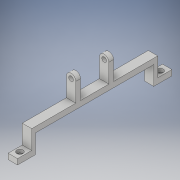
# Autodesk Inventor part: ventilador emergència inferior
Saved by Autodesk Inventor 2019 (Build 230136000, 136)
## iProperties
Created: 2018-10-29
Part Number: ventilador emergència inferior
Material: Genérico
Document SubType Name: Modeling
Designer: Albert Garangou Culebras
Density: 1 g/cm^3
Appearance: Valor por defecto
Author: Albert Garangou Culebras
Autodesk Inventor part; units mm, degrees
ref_plane "YZ Plane" through (0, 0, 0) normal (1, 0, 0) x (0, 1, 0)
ref_plane "XZ Plane" through (0, 0, 0) normal (0, 1, 0) x (-1, 0, 0)
ref_plane "XY Plane" through (0, 0, 0) normal (0, 0, 1) x (1, 0, 0)
sketch "Boceto1" plane through (0, 0, 0) normal (0, 1, 0) x (-1, 0, 0)
  line L0 (0, 12) -> (-3, 12)
  line L1 (-3, 12) -> (0, 12)
  line L2 (0, 12) -> (3, 12)
  line L3 (3, 12) -> (3, 9)
  line L4 (3, 9) -> (-3, 9)
  line L5 (-3, 9) -> (-3, 12)
  line L6 (0, -12) -> (-3, -12)
  line L7 (-3, -12) -> (-3, -9)
  line L8 (-3, -9) -> (3, -9)
  line L9 (3, -9) -> (3, -12)
  line L10 (3, -12) -> (-3, -12)
  point P0 (0, 0)
  constraints: 22 end point, 6 perpendicular, 2 point on line, 1 horizontal, 1 vertical
extrude "Extrusión1" add sketch "Boceto1" along normal blind 15
fillet "Empalme1" radius 3 4 edges at (3, 15, 10.5) (-3, 15, 10.5) (3, 15, -10.5) (-3, 15, -10.5)
sketch "Boceto2" plane through (0, 0, 0) normal (0, -1, 0) x (1, 0, 0)
  line L0 (-3, 9) -> (-3, 12) projected
  line L1 (3, -9) -> (3, -12) projected
  line L2 (-3, 12) -> (3, 12)
  line L3 (3, 12) -> (3, -12)
  line L4 (3, -12) -> (-3, -12)
  line L5 (-3, -12) -> (-3, 12)
  line L6 (3, 0) -> (3, -37.5)
  line L7 (3, 0) -> (3, 37.5)
  line L8 (3, 37.5) -> (-3, 37.5)
  line L9 (-3, 37.5) -> (-3, -37.5)
  line L10 (-3, -37.5) -> (3, -37.5)
  point P0 (0, 0)
  dimension "d11" = 37.5
  dimension "d12" = 37.5
  constraints: 18 end point, 3 perpendicular, 3 point on line, 2 parallel, 1 horizontal, 1 midpoint
  measures "d11" distance of L6.start L6.end
  measures "d12" distance of L6.start L7.end
extrude "Extrusión2" add sketch "Boceto2" along normal blind 3.5
sketch "Boceto3" plane through (0, -3.5, 0) normal (0, -1, 0) x (1, 0, 0)
  line L0 (-3, 37.5) -> (-3, -37.5) projected
  line L1 (3, -37.5) -> (3, 37.5) projected
  line L2 (-3, 37.5) -> (3, 37.5)
  line L3 (3, 37.5) -> (3, 40)
  line L4 (3, 40) -> (-3, 40)
  line L5 (-3, 40) -> (-3, 37.5)
  line L6 (-3, -37.5) -> (3, -37.5)
  line L7 (3, -37.5) -> (3, -40)
  line L8 (3, -40) -> (-3, -40)
  line L9 (-3, -40) -> (-3, -37.5)
  point P0 (0, 0)
  dimension "d15" = 2.5
  dimension "d16" = 2.5
  constraints: 16 end point, 5 perpendicular, 1 collinear, 1 horizontal, 1 point on line
  measures "d15" distance of L1.end L3.end
  measures "d16" distance of L1.start L7.end
extrude "Extrusión3" add sketch "Boceto3" along normal blind 12 contours L5 L4 L3 L2 | L6 L7 L8 L9
sketch "Boceto4" plane through (0, -3.5, 0) normal (0, 1, 0) x (1, 0, 0)
  line L0 (3, -40) -> (-3, -40) projected
  line L1 (3, 37.5) -> (3, -37.5) projected
  line L2 (-3, -40) -> (3, -40)
  line L3 (3, -40) -> (3, -37.5)
  line L4 (3, -37.5) -> (-3, -37.5)
  line L5 (-3, -37.5) -> (-3, -40)
  line L6 (-3, -37.5) -> (-3, 37.5) projected
  line L7 (-3, 40) -> (3, 40) projected
  line L8 (-3, 37.5) -> (3, 37.5)
  line L9 (3, 37.5) -> (3, 40)
  line L10 (3, 40) -> (-3, 40)
  line L11 (-3, 40) -> (-3, 37.5)
  point P0 (0, 0)
  constraints: 16 end point, 4 parallel, 2 horizontal, 2 perpendicular
extrude "Extrusión4" add sketch "Boceto4" along normal blind 3.5 contours L0 L5 L4 L3 | L8 L11 L7 L9
sketch "Boceto5" plane through (-3, -15.5, 40) normal (0, 0, 1) x (1, 0, 0)
  line L0 (0, 0) -> (6, 0) projected
  line L1 (0, 15.5) -> (0, 0) projected
  line L2 (6, 0) -> (0, 0)
  line L3 (0, 0) -> (0, 3.5)
  line L4 (0, 3.5) -> (6, 3.5)
  line L5 (6, 3.5) -> (6, 0)
  point P0 (3, 15.5)
  dimension "d21" = 3.5
  constraints: 8 end point, 2 parallel, 1 horizontal, 1 perpendicular, 1 point on line
  measures "d21" distance of L2.end L3.end
extrude "Extrusión5" add sketch "Boceto5" along normal blind 9
sketch "Boceto6" plane through (3, -15.5, -40) normal (0, 0, -1) x (-1, 0, 0)
  line L0 (6, 0) -> (0, 0) projected
  line L1 (0, 12) -> (0, 0) projected
  line L2 (6, 0) -> (0, 0)
  line L3 (0, 0) -> (0, 3.5)
  line L4 (0, 3.5) -> (6, 3.5)
  line L5 (6, 3.5) -> (6, 0)
  point P0 (3, 15.5)
  dimension "d24" = 3.5
  constraints: 8 end point, 2 parallel, 1 horizontal, 1 perpendicular, 1 point on line
  measures "d24" distance of L2.end L3.end
extrude "Extrusión6" add sketch "Boceto6" along normal blind 9
sketch "Boceto7" plane through (0, 12, 12) normal (0, 0, 1) x (1, 0, 0)
  circle A0 centre (0, 0) radius 1.5
  point P0 (0, -12)
  dimension "d27" = 3
  constraints: 1 centre point
  measures "d27" diameter of A0
extrude "Extrusión7" cut sketch "Boceto7" against normal blind 31.25
sketch "Boceto8" plane through (-3, -12, 40) normal (0, 1, 0) x (1, 0, 0)
  line L0 (0, -9) -> (6, -9) projected
  line L1 (3, -9) -> (3, 0)
  line L2 (0, 0) -> (6, 0) projected
  line L3 (3, -4.5) -> (4.913, -4.5)
  line L4 (6, 80) -> (0, 80) projected
  line L5 (3, 80) -> (3, 89.023)
  line L6 (3, 84.5115) -> (4.913, 84.5115)
  point P0 (3, 40)
  constraints: 8 end point, 5 midpoint, 2 horizontal, 1 vertical
hole "Agujero1" at (0, -12, -44.5115) at (0, -12, 44.5) direction (0, -1, 0) diameter 2.9 depth 10 counterbore diameter 4 counterbore depth 2
